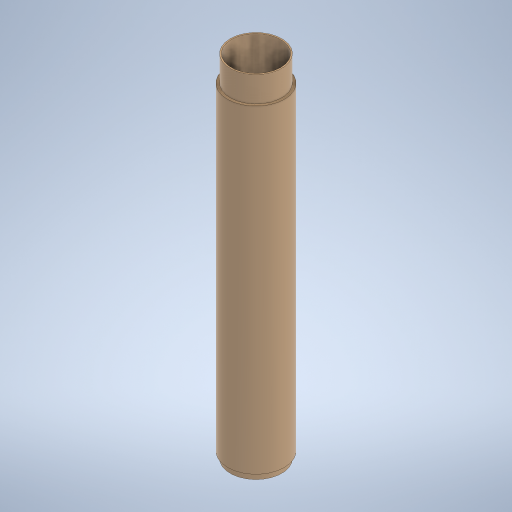
# Autodesk Inventor part: BodyCylinder
Saved by Autodesk Inventor 2024 (Build 280153000, 153)
## iProperties
Created: 2023-09-22
Part Number: BodyCylinder
Material: Brass
Document SubType Name: Modeling
Designer: schanen
Density: 8.49 g/cm^3
Appearance: Brindle
Author: schanen
Autodesk Inventor part; units mm, degrees
ref_plane "YZ Plane" through (0, 0, 0) normal (1, 0, 0) x (0, 1, 0)
ref_plane "XZ Plane" through (0, 0, 0) normal (0, 1, 0) x (-1, 0, 0)
ref_plane "XY Plane" through (0, 0, 0) normal (0, 0, 1) x (1, 0, 0)
sketch "Sketch1" plane through (0, 0, 0) normal (0, 0, 1) x (1, 0, 0)
  line L0 (-19.225, 0) -> (-22.225, 0)
  line L1 (-22.225, 0) -> (-22.225, 250)
  line L2 (-22.225, 250) -> (-19.225, 250)
  line L3 (-19.225, 250) -> (-19.225, 0)
  line L4 (0, -60) -> (0, 325) projected
  line L5 (-19.225, 250) -> (-20.225, 250)
  line L6 (-20.225, 250) -> (-20.225, 270)
  line L7 (-20.225, 270) -> (-19.225, 270)
  line L8 (-19.225, 270) -> (-19.225, 250)
  line L9 (-19.225, 0) -> (-20.225, 0)
  line L10 (-20.225, 0) -> (-20.225, -5)
  line L11 (-20.225, -5) -> (-19.225, -5)
  line L12 (-19.225, -5) -> (-19.225, 0)
  point P0 (0, 0)
  point P1 (-20.225, 0)
  dimension "d0" = 22.225
  dimension "d1" = 3
  dimension "d2" = 250
  dimension "d4" = 1
  dimension "d5" = 20
  dimension "d6" = 1
  dimension "d7" = 5
  constraints: 24 end point, 6 parallel, 3 horizontal, 3 perpendicular, 1 horizontal alignment
  measures "d0" distance from line of point (0, 0) L1
  measures "d1" distance between parallel lines of L3 L1
  measures "d2" distance of L0.end L1.end
  measures "d4" distance of L6.end L7.end
  measures "d5" distance of L5.end L6.end
  measures "d6" distance of L11.end L10.end
  measures "d7" distance of L10.end L9.end
revolve "Revolution1" add sketch "Sketch1" angle 360 about axis through (0, -10, 0) along (0, 1, 0)
body "Solid1"
